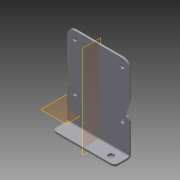
# Autodesk Inventor part: Pneumatics_VIAIR_0090_01
Saved by Autodesk Inventor 2014 (Build 180170000, 170)
## iProperties
Created: 2011-02-24
Part Number: Pneumatics_VIAIR_0090_01
Document SubType Name: Modeling
Designer: s-2512184
Density: 2.71 g/cm^3
Material: Aluminum-6061
Mass: 16.1968 g
Surface Area: 79.7048 cm^2
Volume: 5.97666 cm^3
Description: AIR COMPRESSOR MOUNT 2
Vendor: VIAIR
Appearance: Aluminum - Flat
Author: s-2512184
Title: AIR COMPRESSOR MOUNT 2
Autodesk Inventor part; units mm, degrees
ref_plane "XZ Plane" through (0, 0, 0) normal (0, 1, 0) x (-1, 0, 0)
ref_plane "XY Plane" through (0, 0, 0) normal (0, 0, 1) x (1, 0, 0)
sketch "Sketch1" plane through (0, 0, 0) normal (0, 0, 1) x (1, 0, 0)
  line L0 (-26.797, 31.75) -> (26.797, 31.75)
  line L1 (26.797, 31.75) -> (26.797, -31.75)
  line L2 (26.797, -31.75) -> (-26.797, -31.75)
  line L3 (-26.797, -31.75) -> (-26.797, 31.75)
  point P0 (0, 0)
  point P1 (-26.797, 0)
  point P2 (0, 31.75)
  dimension "d0" = 53.594
  dimension "d1" = 63.5
  constraints: 8 end point, 2 midpoint, 2 parallel, 1 horizontal, 1 horizontal alignment, 1 perpendicular, 1 vertical alignment
  measures "d0" distance of L1.end L2.end
  measures "d1" distance of L2.end L0.start
extrude "Extrusion1" add sketch "Sketch1" along normal blind 1.5875
sketch "Sketch9" plane through (0, 0, 1.5875) normal (0, 0, 1) x (1, 0, 0)
  line L0 (26.797, 31.75) -> (26.797, -31.75) projected
  line L1 (-26.797, -31.75) -> (-26.797, 31.75) projected
  line L2 (26.797, -31.75) -> (-26.797, -31.75) projected
  line L3 (-26.797, -31.75) -> (26.797, -31.75)
  line L4 (26.797, -31.75) -> (26.797, -40.7924)
  line L5 (26.797, -40.7924) -> (-26.797, -40.7924)
  line L6 (-26.797, -40.7924) -> (-26.797, -31.75)
  line L7 (-26.797, 31.75) -> (26.797, 31.75) projected
  point P0 (0, 0)
  dimension "d60" = 72.5424
  constraints: 8 end point, 2 collinear, 2 parallel, 1 horizontal, 1 perpendicular, 1 point on line
  measures "d60" distance between parallel lines of L5 L7
extrude "Extrusion5" add sketch "Sketch9" against normal up to surface (1.5875 mm away) contours L4 L5 L6 L2
sketch "Sketch2" plane through (0, 0, 1.5875) normal (0, 0, 1) x (1, 0, 0)
  line L0 (-26.797, -39.1922) -> (26.797, -39.1922)
  line L1 (26.797, -40.7924) -> (-26.797, -40.7924)
  line L2 (26.797, -40.7924) -> (26.797, 31.75) projected
  line L3 (-26.797, -40.7924) -> (26.797, -40.7924) projected
  line L4 (-26.797, -40.7924) -> (-26.797, -39.1922)
  line L5 (26.797, -40.7924) -> (26.797, -39.1922)
  point P0 (-26.797, -31.75)
  point P1 (0, 0)
  dimension "d4" = 53.594
  dimension "d59" = 1.6002
  constraints: 8 end point, 2 collinear, 1 horizontal, 1 parallel, 1 perpendicular
  measures "d4" distance of L1.end L1.start
  measures "d59" distance between parallel lines of L0 L1
extrude "Extrusion2" add sketch "Sketch2" along normal blind 12.7
sketch "Sketch6" plane through (0, 0, 1.5875) normal (0, 0, 1) x (1, 0, 0)
  line L0 (26.797, 31.75) -> (26.797, -29.3687) projected
  line L1 (-26.797, 31.75) -> (26.797, 31.75) projected
  line L2 (-26.797, -29.3687) -> (-26.797, 31.75) projected
  arc A0 (20.447, -21.844) -> (23.9286, -10.1836) centre (20.447, -15.494) ccw projected
  arc A1 (23.4121, -8.0836) -> (23.9286, -10.1836) centre (24.799, -8.856) ccw projected
  arc A2 (23.4121, -8.0836) -> (26.797, 4.953) centre (0, 4.953) ccw projected
  line L3 (26.797, 25.4) -> (26.797, 4.953) projected
  arc A3 (26.797, 25.4) -> (20.447, 31.75) centre (20.447, 25.4) ccw projected
  line L4 (14.199, 31.75) -> (20.447, 31.75) projected
  line L5 (-14.199, 31.75) -> (14.199, 31.75) projected
  line L6 (-20.447, 31.75) -> (-14.199, 31.75) projected
  arc A4 (-20.447, 31.75) -> (-26.797, 25.4) centre (-20.447, 25.4) ccw projected
  line L7 (-26.797, 4.953) -> (-26.797, 25.4) projected
  arc A5 (-26.797, 4.953) -> (-23.4121, -8.0836) centre (0, 4.953) ccw projected
  arc A6 (-23.9286, -10.1836) -> (-23.4121, -8.0836) centre (-24.799, -8.856) ccw projected
  arc A7 (-23.9286, -10.1836) -> (-20.447, -21.844) centre (-20.447, -15.494) ccw projected
  line L8 (20.447, -21.844) -> (-20.447, -21.844) projected
  arc A8 (-23.9286, -10.1836) -> (-26.797, -15.494) centre (-20.447, -15.494) ccw
  arc A9 (26.797, -15.494) -> (23.9286, -10.1836) centre (20.447, -15.494) ccw
  arc A10 (23.4121, -8.0836) -> (23.9286, -10.1836) centre (24.799, -8.856) ccw
  arc A11 (-23.9286, -10.1836) -> (-23.4121, -8.0836) centre (-24.799, -8.856) ccw
  point P0 (0, 0)
  constraints: 10 point on circle, 4 centre point, 4 coincident, 4 concentric, 2 end point, 2 point on line
extrude "Extrusion4" cut sketch "Sketch6" against normal up to next contours L0 A3 L1 | L0 A0 A1 A2 | A4 L2 L1 | L2 A5 A6 A7
sketch "Sketch7" plane through (0, 0, 1.5875) normal (0, 0, 1) x (1, 0, 0)
  arc A0 (26.797, 25.4) -> (20.447, 31.75) centre (20.447, 25.4) ccw projected
  arc A1 (-20.447, 31.75) -> (-26.797, 25.4) centre (-20.447, 25.4) ccw projected
  arc A2 (-23.9286, -10.1836) -> (-26.797, -15.494) centre (-20.447, -15.494) ccw projected
  arc A3 (26.797, -15.494) -> (23.9286, -10.1836) centre (20.447, -15.494) ccw projected
  point P0 (0, 0)
hole "Hole3" at (-20.447, 25.4, 1.5875) at (20.447, 25.4, 1.5875) at (20.447, -15.494, 1.5875) at (-20.447, -15.494, 1.5875) direction (0, 0, -1) diameter 3.81 end through all clearance for "Oval Head Machine Screw" size "#6" standard "Ansi Unified Screw Threads"
ref_plane "Work Plane1" through (-26.797, -30.1625, 2.3812) normal (0, 1, 0) x (1, 0, 0)
fillet "Fillet3" radius 1.6002 1 edges at (0, -39.1922, 1.5875)
fillet "Fillet4" radius 3.175 1 edges at (0, -40.7924, 0)
fillet "Fillet5" radius 3.175 2 edges at (-26.797, -39.9923, 14.2875) (26.797, -39.9923, 14.2875)
sketch "Sketch10" plane through (-26.797, -39.1922, 3.1877) normal (0, 1, 0) x (1, 0, 0)
  circle A0 centre (44.831, -5.4264) radius 2.4116 projected
  point P0 (26.797, 3.1877)
hole "Hole6" at (18.034, -39.1922, 8.6141) direction (0, -1, 0) diameter 5.1054 end through all clearance for "Flat Head Machine Screw (82)" size "#10" standard "Ansi Unified Screw Threads"
mirror "Mirror1" about plane through (0, 0, 0) normal (1, 0, 0) of "Hole6"
body "Solid1"
